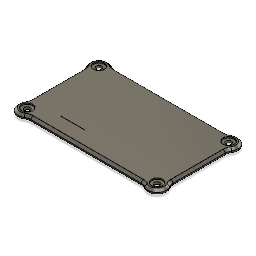
Baseplate-lobed (Autodesk Fusion 360 design; units mm, degrees)
Autodesk Fusion 360 part; units mm, degrees
sketch "face" plane through (0, 0, 0) normal (0, 1, 0) x (1, 0, 0)
  line L0 (13, -14.3) -> (-13, -14.3)
  line L1 (-13, -14.3) -> (-13, 14.3)
  line L2 (-13, 14.3) -> (13, 14.3)
  line L3 (13, 14.3) -> (13, -14.3)
  line L4 (13, -14.3) -> (-13, 14.3) construction
  line L5 (-13, -14.3) -> (13, 14.3) construction
  line L6 (-9, 12.22) -> (9, 12.22)
  line L7 (0, 18) -> (0, -18)
  line L8 (-10, 14.3) -> (-7, 14.3)
  line L9 (-7, 14.3) -> (-7, 17.3)
  line L10 (-7, 17.3) -> (-10, 17.3)
  line L11 (-10, 17.3) -> (-10, 14.3)
  line L12 (7, 14.3) -> (7, 17.3)
  line L13 (7, 17.3) -> (10, 17.3)
  line L14 (10, 17.3) -> (10, 14.3)
  line L15 (10, 14.3) -> (7, 14.3)
  line L16 (-20, -0.0009) -> (20, -0.0009)
  line L17 (-7, -17.3017) -> (-10, -17.3017)
  line L18 (-10, -17.3017) -> (-10, -14.3017)
  line L19 (-7, -14.3017) -> (-7, -17.3017)
  line L20 (-10, -14.3017) -> (-7, -14.3017)
  line L21 (7, -17.3017) -> (10, -17.3017)
  line L22 (7, -14.3017) -> (7, -17.3017)
  line L23 (10, -17.3017) -> (10, -14.3017)
  line L24 (10, -14.3017) -> (7, -14.3017)
  line L25 (-7, 14.3) -> (6, 14.3)
  line L26 (6, 14.3) -> (6, 12.7854)
  line L27 (6, 12.7854) -> (-7, 12.7854)
  line L28 (-7, 12.7854) -> (-7, 14.3)
  line L29 (-7, -14.3017) -> (6, -14.3017)
  line L30 (6, -14.3017) -> (6, -12)
  line L31 (6, -12) -> (-7, -12)
  line L32 (-7, -12) -> (-7, -14.3017)
  line L33 (-13, 14.3) -> (-15, 14.3)
  line L34 (-15, 14.3) -> (-15, -14.3)
  line L35 (-15, -14.3) -> (-13, -14.3)
  line L36 (-13, -14.3) -> (-13, 14.3)
  line L37 (13, 14.3) -> (15, 14.3)
  line L38 (15, 14.3) -> (15, -14.3)
  line L39 (15, -14.3) -> (13, -14.3)
  line L40 (13, -14.3) -> (13, 14.3)
  line L41 (45, 23) -> (45, -32)
  circle A0 centre (-20, -19.3) radius 3
  circle A1 centre (-20, -19.3) radius 1.5
  circle A2 centre (50, -19.3) radius 3
  circle A3 centre (50, -19.3) radius 1.5
  circle A4 centre (-20, 19.2983) radius 3
  circle A5 centre (-20, 19.2983) radius 1.5
  circle A6 centre (50, 19.2983) radius 3
  circle A7 centre (50, 19.2983) radius 1.5
  line L42 (-25, 24.2983) -> (55, 24.2983)
  line L43 (55, 24.2983) -> (55, -24.3)
  line L44 (55, -24.3) -> (-25, -24.3)
  line L45 (-25, -24.3) -> (-25, 24.2983)
  line L46 (-7, -14.3017) -> (-6, -14.3017)
  line L47 (-6, -14.3017) -> (-6, -12)
  line L48 (-6, -12) -> (-7, -12)
  line L49 (-7, -12) -> (-7, -14.3017)
  line L50 (-7, 14.3) -> (-5.9976, 14.3)
  line L51 (-5.9976, 14.3) -> (-5.9976, 12.7854)
  line L52 (-5.9976, 12.7854) -> (-7, 12.7854)
  line L53 (-7, 12.7854) -> (-7, 14.3)
  line L54 (36, 10.72) -> (24, -1.28) construction
  line L55 (24, 10.72) -> (36, -1.28) construction
  line L56 (25, 5.72) -> (23, 3.72) construction
  line L57 (23, 5.72) -> (25, 3.72) construction
  line L58 (44.7322, -22.8) -> (-14.7322, -22.8)
  line L59 (-23.5, -14.0322) -> (-23.5, 14.0305)
  line L60 (-14.7322, 22.7983) -> (44.7322, 22.7983)
  line L61 (53.5, 14.0305) -> (53.5, -14.0322)
  arc A8 (-17.3661, 23.5483) -> (-24.25, 16.6644) centre (-20, 19.2983) ccw
  arc A9 (-23.5, 15.7276) -> (-16.4293, 22.7983) centre (-20, 19.2983) ccw
  arc A10 (54.25, 16.6644) -> (47.3661, 23.5483) centre (50, 19.2983) ccw
  arc A11 (46.4293, 22.7983) -> (45, 19.2983) centre (50, 19.2983) ccw
  arc A12 (45, 19.2983) -> (53.5, 15.7276) centre (50, 19.2983) ccw
  arc A13 (53.5, -15.7293) -> (45, -19.3) centre (50, -19.3) ccw
  arc A14 (45, -19.3) -> (46.4293, -22.8) centre (50, -19.3) ccw
  arc A15 (50, -24.3) -> (54.25, -16.6661) centre (50, -19.3) ccw
  arc A16 (47.3661, -23.55) -> (50, -24.3) centre (50, -19.3) ccw
  arc A17 (-24.25, -16.6661) -> (-20, -24.3) centre (-20, -19.3) ccw
  arc A18 (-20, -24.3) -> (-17.3661, -23.55) centre (-20, -19.3) ccw
  arc A19 (-16.4293, -22.8) -> (-23.5, -15.7293) centre (-20, -19.3) ccw
  arc A20 (-17.3661, 23.5483) -> (-14.7322, 22.7983) centre (-14.7322, 27.7983) ccw
  arc A21 (-23.5, 14.0305) -> (-24.25, 16.6644) centre (-28.5, 14.0305) ccw
  arc A22 (44.7322, 22.7983) -> (47.3661, 23.5483) centre (44.7322, 27.7983) ccw
  arc A23 (54.25, 16.6644) -> (53.5, 14.0305) centre (58.5, 14.0305) ccw
  arc A24 (53.5, -14.0322) -> (54.25, -16.6661) centre (58.5, -14.0322) ccw
  arc A25 (47.3661, -23.55) -> (44.7322, -22.8) centre (44.7322, -27.8) ccw
  arc A26 (-14.7322, -22.8) -> (-17.3661, -23.55) centre (-14.7322, -27.8) ccw
  arc A27 (-24.25, -16.6661) -> (-23.5, -14.0322) centre (-28.5, -14.0322) ccw
  arc A28 (-23.5, 14.0305) -> (-24.25, 16.6644) centre (-28.5, 14.0305) ccw
  line L62 (-10.5289, 15.75) -> (10.2671, 15.75) construction
  line L63 (10.2671, 15.75) -> (10.2671, 19.75) construction
  line L64 (10.2671, 19.75) -> (-10.5289, 19.75) construction
  line L65 (-10.5289, 19.75) -> (-10.5289, 15.75) construction
  line L66 (51.5, -20.8) -> (-21.5, -20.8)
  line L67 (-21.5, -20.8) -> (-21.5, 20.7983)
  line L68 (-21.5, 20.7983) -> (51.5, 20.7983)
  line L69 (51.5, 20.7983) -> (51.5, -20.8)
  line L70 (-20, 19.2983) -> (50, 19.2983)
  line L71 (50, 19.2983) -> (50, -19.3)
  line L72 (50, -19.3) -> (-20, -19.3)
  line L73 (-20, -19.3) -> (-20, 19.2983)
  point P0 (30, 4.72)
  point P1 (24, 4.72)
  dimension "d1" = 26
  dimension "d2" = 28.6
  dimension "d4" = 18
  dimension "d5" = 2.08
  dimension "d8" = 3
  dimension "d9" = 3
  dimension "d10" = 3
  dimension "d11" = 3
  dimension "d12" = 2
  dimension "d13" = 2
  dimension "d19" = 15
  dimension "d20" = 15
  dimension "d21" = 6
  dimension "d22" = 3
  dimension "d23" = 5
  dimension "d24" = 5
  dimension "d25" = 5
  dimension "d26" = 5
  dimension "d27" = 5
  dimension "d28" = 5
  dimension "d47" = 12
  dimension "d48" = 12
  dimension "d51" = 2
  dimension "d52" = 2
  dimension "d55" = 10
  dimension "d56" = 10
  dimension "d57" = 10
  dimension "d58" = 10
  dimension "d61" = 5
  dimension "d62" = 5
  dimension "d63" = 5
  dimension "d64" = 5
  dimension "d65" = 5
  dimension "d66" = 5
  dimension "d67" = 5
  dimension "d68" = 5
  dimension "d69" = 5
  dimension "d74" = 3.5
  dimension "d75" = 5
  measures "d1" distance of L1.end L2.end
  measures "d2" distance of L0.end L1.end
  measures "d4" distance of L6.start L6.end
  measures "d5" distance of L2 L6
  measures "d8" distance of L8.start L8.end
  measures "d9" distance of L8.start L10.end
  measures "d10" distance of L1.end L8.start
  measures "d11" distance of L2.end L14.end
  measures "d12" distance of L1.end L33.end
  measures "d13" distance of L2.end L37.end
  measures "d19" distance of L38 P0
  measures "d20" distance of L41 P0
  measures "d21" diameter of A0
  measures "d22" diameter of A1
  measures "d23" distance of L34.end A0.centre
  measures "d24" distance of L35 A0.centre
  measures "d25" distance of A4.centre L45
  measures "d26" distance of A4.centre L42
  measures "d27" distance of A6.centre L43
  measures "d28" distance of A2.centre L44
  measures "d47" distance of L54.end L55.end
  measures "d48" distance of L55.start L54.end
  measures "d51" distance of L56.end L57.end
  measures "d52" distance of L57.start L56.end
  measures "d55" diameter of A8
  measures "d56" diameter of A17
  measures "d57" diameter of A14
  measures "d58" diameter of A10
  measures "d61" radius of A20
  measures "d62" radius of A21
  measures "d63" radius of A22
  measures "d64" radius of A23
  measures "d65" radius of A24
  measures "d66" radius of A25
  measures "d67" radius of A26
  measures "d68" radius of A27
  measures "d69" radius of A28
extrude "Extrude11" add sketch "face" against normal blind 1.5 contours L41 A9 L68 L70 | L41 A19 L66 L72 | A12 A13 L69 L71 | A9 A19 L67 L73 makes body 1 at (-21.5, -0.5, 4.844) makes body 2 at (4.8465, -0.5, -20.7983) makes body 3 at (24.9232, -1, 20.8) makes body 4 at (51.5, -0.5, -4.8423)
extrude "Extrude3" add sketch "face" along normal blind 2 separate body contours L17 L18 L19 L20 | L0 L3 L7 L16 L30 L31 L40 | L3 L16 L38 L39 L40 | L0 L7 L30 L31 | L2 L3 L7 L15 L16 L26 L27 L40 | L3 L16 L37 L38 L40 | L0 L7 L31 L47 | L1 L2 L7 L8 L16 L27 L28 L36 L52 L53 | L0 L1 L7 L16 L31 L32 L36 L48 L49 | L0 L31 L32 L47 L48 L49 | L2 L12 L13 L14 L15 | L1 L16 L33 L34 L36 | L1 L16 L34 L35 L36 | L2 L7 L25 L27 L51 | L2 L7 L25 L26 L27 | L2 L25 L27 L28 L50 L51 L52 L53 | L2 L8 L9 L10 L11 | L21 L22 L23 L24 | L41 A12 A13 L71 | L41 A9 L68 L70 | L41 A11 L68 | A6 A12 L70 L71 | L41 A9 A19 L70 L72 L73 | A6 A11 L68 L70 | L41 A14 L66 | A2 A14 L66 L72 | A2 A13 L71 L72 | L41 A19 L66 L72 | L41 A0 A4 L58 L59 L60 A8 A17 A18 A20 A21 A22 A25 A26 A27 A28 L66 L67 L68 | L41 A2 A6 L61 A10 A15 A16 A22 A23 A24 A25 L66 L68 L69 | A6 A12 L69 L71 | A12 A13 L69 L71 | A4 A9 L68 L70 | A4 A9 L70 L73 | A6 A7 L70 L71 | A6 A7 L68 L70 | A2 A13 L69 L71 | A2 A3 L66 L72 | A2 A3 L71 L72 | A0 A19 L72 L73 | A0 A19 L66 L72 | A6 L68 L69 | A6 A7 L69 L71 | A9 A19 L67 L73 | A4 A9 L67 L73 | A4 A5 L68 L70 | A4 A5 L70 L73 | A2 A3 L69 L71 | A2 L66 L69 | A0 A19 L67 L73 | A0 A1 L72 L73 | A0 A1 L66 L72 | A4 L67 L68 | A7 L68 L69 | A4 A5 L67 L73 | A0 L66 L67 | A3 L66 L69 | A0 A1 L67 L73 | A5 L67 L68 | A1 L66 L67 makes body 5
extrude "Extrude4" add sketch "face" along normal blind 0.7 separate body contours A6 A7 L70 L71 | A6 A7 L68 L70 | A2 A3 L66 L72 | A2 A3 L71 L72 | A6 L68 L69 | A6 A7 L69 L71 | A4 A5 L68 L70 | A4 A5 L70 L73 | A2 A3 L69 L71 | A2 L66 L69 | A0 A1 L72 L73 | A0 A1 L66 L72 | A4 L67 L68 | A7 L68 L69 | A4 A5 L67 L73 | A0 L66 L67 | A3 L66 L69 | A0 A1 L67 L73 | A5 L67 L68 | A1 L66 L67 makes body 6 at (-17.5112, 0.7, -19.4473) makes body 7 at (52.4832, 0.7, 19.0764) makes body 8 at (-17.5168, 0.7, 19.0764) makes body 9 at (52.4832, 0, -19.0747)
move_body "Move1" bodies 9 8 7 6 to x (1, 0, 0) y (0, 1, 0) z (0, 0, 1) at (0, 1.3, 0)
combine "Combine1" operation cut target body 5 tool bodies 9 8 7 6
chamfer "Chamfer6" distance 1.2 angle 45 16 edges at (-23.5355, 2, -22.8338) (-23.6912, 2, -15.3998) (-23.5, 2, 0.0009) (-23.6912, 2, 15.4015) (-23.5355, 2, 22.8355) (-16.1015, 2, 22.9912) (15, 2, 22.8) (46.1015, 2, 22.9912) (53.5355, 2, 22.8355) (53.6912, 2, 15.4015) (53.5, 2, 0.0009) (53.6912, 2, -15.3998) (53.5355, 2, -22.8338) (46.1015, 2, -22.9895) (15, 2, -22.7983) (-16.1015, 2, -22.9895) on bodies 5
combine "Combine14" operation add target body 5 tool bodies 1 4 3 2
named bodies: "Baseplate"
